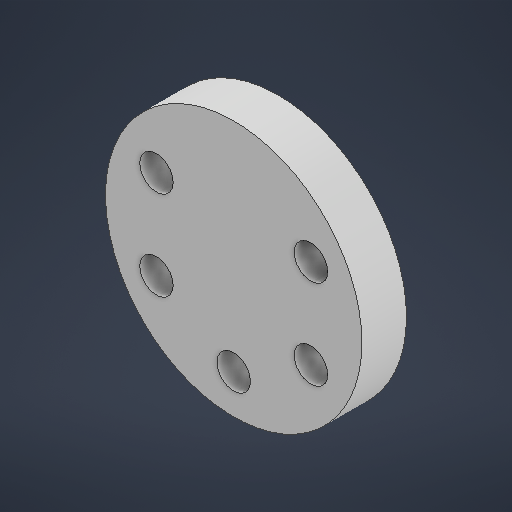
# Autodesk Inventor part: проставка шкив стреляло
Saved by Autodesk Inventor 2026.2 (Build 302298000, 298)
## iProperties
Created: 2025-12-13
Part Number: проставка шкив стреляло
Material: Типовые
Document SubType Name: Modeling
Designer: Phantom
Density: 1 g/cm^3
Appearance: По умолчанию
Author: Phantom
Autodesk Inventor part; units mm, degrees
ref_plane "YZ Plane" through (0, 0, 0) normal (1, 0, 0) x (0, 1, 0)
ref_plane "XZ Plane" through (0, 0, 0) normal (0, 1, 0) x (-1, 0, 0)
ref_plane "XY Plane" through (0, 0, 0) normal (0, 0, 1) x (1, 0, 0)
sketch "Эскиз1" plane through (0, 0, 0) normal (0, 0, 1) x (1, 0, 0)
  circle A0 centre (-7.1186, 4.4733) radius 1.25
  circle A1 centre (-7.1186, -3.5267) radius 1.25
  circle A2 centre (-0.1904, 0.4733) radius 4.925
  circle A3 centre (-0.1904, -7.5267) radius 1.25
  circle A4 centre (6.7378, -3.5267) radius 1.25
  circle A5 centre (6.7378, 4.4733) radius 1.25
  circle A6 centre (-7.1186, 4.4733) radius 1.5
  circle A7 centre (-0.1904, 0.4733) radius 11.5
  circle A8 centre (-7.1186, -3.5267) radius 1.5
  circle A9 centre (-0.1904, -7.5267) radius 1.5
  circle A10 centre (6.7378, -3.5267) radius 1.5
  circle A11 centre (6.7378, 4.4733) radius 1.5
  point P0 (0, 0)
  dimension "d0" = 3
  dimension "d1" = 23
  dimension "d2" = 3
  dimension "d3" = 3
  dimension "d4" = 3
  dimension "d5" = 3
  constraints: 12 centre point, 5 coincident
  measures "d0" diameter of A6
  measures "d1" diameter of A7
  measures "d2" diameter of A8
  measures "d3" diameter of A9
  measures "d4" diameter of A10
  measures "d5" diameter of A11
extrude "Выдавливание1" add sketch "Эскиз1" along normal blind 4 contours A2 | A7
